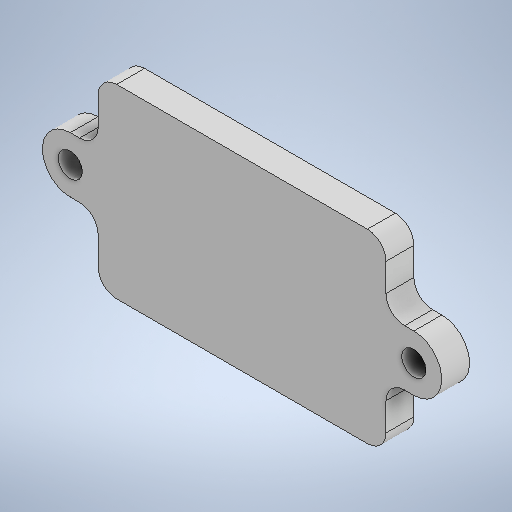
# Autodesk Inventor part: ude_sensor
Saved by Autodesk Inventor 2025.1 (Build 291241000, 241)
## iProperties
Created: 2024-09-09
Part Number: ude_sensor
Material: 一般
Document SubType Name: Modeling
Designer: right
Density: 1 g/cm^3
Appearance: 既定
Author: right
Autodesk Inventor part; units mm, degrees
ref_plane "YZ Plane" through (0, 0, 0) normal (1, 0, 0) x (0, 1, 0)
ref_plane "XZ Plane" through (0, 0, 0) normal (0, 1, 0) x (-1, 0, 0)
ref_plane "XY Plane" through (0, 0, 0) normal (0, 0, 1) x (1, 0, 0)
sketch "スケッチ1" plane through (0, 0, 0) normal (0, 0, 1) x (1, 0, 0)
  line L0 (0, 0) -> (0, 2.6709) construction
  circle A0 centre (-18.5, 0) radius 1.3
  circle A1 centre (18.5, 0) radius 1.3
  circle A2 centre (-18.5, 0) radius 3
  circle A3 centre (18.5, 0) radius 3
  line L1 (-18.5, 3) -> (18.5, 3)
  line L2 (-18.5, -3) -> (18.5, -3)
  line L3 (-15.5, 10) -> (15.5, 10)
  line L4 (15.5, 10) -> (15.5, -10)
  line L5 (15.5, -10) -> (-15.5, -10)
  line L6 (-15.5, -10) -> (-15.5, 10)
  point P0 (-18.5, 3)
  point P1 (15.5, -3)
  point P2 (-15.5, -3)
  point P3 (-15.5, 3)
  point P4 (15.5, 3)
  dimension "d0" = 2.6
  dimension "d1" = 18.5
  dimension "d2" = 6
  dimension "d3" = 6
  dimension "d6" = 7
  dimension "d7" = 7
  constraints: 14 end point, 6 tangent, 4 centre point, 4 point on circle, 2 coincident, 2 parallel, 1 horizontal, 1 horizontal alignment, 1 perpendicular, 1 symmetric about line, 1 vertical, 1 other
  measures "d0" diameter of A0
  measures "d1" distance from line of L0 A0.centre
  measures "d2" diameter of A2
  measures "d3" diameter of A3
  measures "d6" distance from line of L1.end L3
  measures "d7" distance from line of L2.end L5
extrude "押し出し1" add sketch "スケッチ1" along normal blind 3
fillet "フィレット1" radius 2 8 edges at (-15.5, 3, 1.5) (-15.5, -3, 1.5) (15.5, 3, 1.5) (15.5, -3, 1.5) (-15.5, -10, 1.5) (-15.5, 10, 1.5) (15.5, 10, 1.5) (15.5, -10, 1.5)
equation "\"d7\" = d6"
